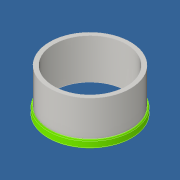
# Autodesk Inventor part: CoverBase
Saved by Autodesk Inventor 2016 (Build 200138000, 138)
## iProperties
Created: 2015-08-24
Part Number: CoverBase
Material: ABS-Kunststoff
Document SubType Name: Modeling
Designer: 4ndreas
Density: 1.06 g/cm^3
Appearance: Glatt - grün
Author: 4ndreas
Autodesk Inventor part; units mm, degrees
ref_plane "YZ Plane" through (0, 0, 0) normal (1, 0, 0) x (0, 1, 0)
ref_plane "XZ Plane" through (0, 0, 0) normal (0, 1, 0) x (-1, 0, 0)
ref_plane "XY Plane" through (0, 0, 0) normal (0, 0, 1) x (1, 0, 0)
sketch "Skizze1" plane through (0, 0, 0) normal (0, 0, 1) x (1, 0, 0)
  line L0 (-69.282, 40) -> (69.282, 40) projected
  arc A0 (69.282, -40) -> (80, 0) centre (0, 0) ccw projected
  arc A1 (80, 0) -> (69.282, 40) centre (0, 0) ccw projected
  circle A2 centre (-61.0246, -30) radius 2.25 projected
  circle A3 centre (-61.0246, 30) radius 2.25 projected
  circle A4 centre (68, 0) radius 2.25 projected
  circle A5 centre (61.0246, 30) radius 2.25 projected
  circle A6 centre (61.0246, -30) radius 2.25 projected
  circle A7 centre (-68, 0) radius 2.25 projected
  line L1 (59.925, 53) -> (-59.925, 53) projected
  arc A8 (59.925, 53) -> (-59.925, 53) centre (0, 0) ccw projected
  line L2 (59.925, 53) -> (-59.925, 53) projected
  arc A9 (-59.925, 53) -> (-69.282, 40) centre (0, 0) ccw projected
  line L3 (-69.282, 40) -> (69.282, 40) projected
  arc A10 (69.282, 40) -> (59.925, 53) centre (0, 0) ccw projected
  circle A11 centre (0, 0) radius 83
  line L4 (69.282, -40) -> (-69.282, -40) projected
  arc A12 (-69.282, 40) -> (-69.282, -40) centre (0, 0) ccw projected
  circle A13 centre (0, 0) radius 80
  point P0 (0, 0)
  dimension "d0" = 3
  constraints: 2 centre point, 2 coincident, 1 concentric
  measures "d0" radial gap between concentric circles of A8 A11
extrude "Extrusion1" add sketch "Skizze1" against normal blind 10 contours A11
sketch "Skizze3" plane through (0, 0, -10) normal (0, 0, -1) x (-1, 0, 0)
  circle A0 centre (0, 0) radius 83 projected
  circle A1 centre (0, 0) radius 72
  circle A2 centre (0, 0) radius 80 projected
  circle A3 centre (0, 0) radius 83 projected
  point P0 (0, 0)
  dimension "d11" = 11
  constraints: 1 centre point, 1 coincident
  measures "d11" radial gap between concentric circles of A0 A1
extrude "Extrusion2" add sketch "Skizze3" against normal blind 80 separate body contours A2
sketch "Skizze4" plane through (0, 0, -10) normal (0, 0, -1) x (-1, 0, 0)
  circle A0 centre (0, 0) radius 83 projected
  circle A1 centre (0, 0) radius 80 projected
  circle A2 centre (0, 0) radius 83 projected
  point P0 (0, 0)
extrude "Extrusion3" add sketch "Skizze4" along normal blind 5 bodies 1
fillet "Rundung1" radius 2 2 edges at (83, 0, -15) (-83, 0, 0)
